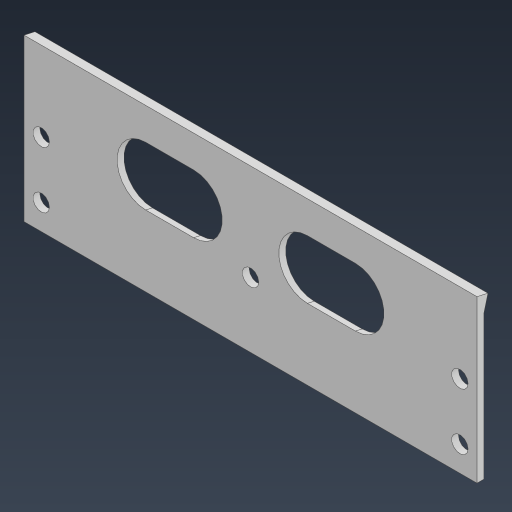
# Autodesk Inventor part: plastic_front
Saved by Autodesk Inventor 2023 (Build 270158000, 158)
## iProperties
Created: 2026-01-11
Part Number: plastic_front
Material: Generic
Document SubType Name: Modeling
Designer: szymo
Density: 14.3899 g/cm^3
Appearance: Default
Mass: 65 g
Surface Area: 65.7357 cm^2
Volume: 4.51705 cm^3
Author: szymo
Autodesk Inventor part; units mm, degrees
ref_plane "YZ Plane" through (0, 0, 0) normal (1, 0, 0) x (0, 1, 0)
ref_plane "XZ Plane" through (0, 0, 0) normal (0, 1, 0) x (-1, 0, 0)
ref_plane "XY Plane" through (0, 0, 0) normal (0, 0, 1) x (1, 0, 0)
ref_plane "Work Plane1" through (0, -9.9648, -37.8181) normal (-1, 0, 0) x (0, 0.2547957, 0.9669949)
sketch "Sketch1" plane through (0, -9.9648, -37.8181) normal (-1, 0, 0) x (0, 0.2547957, 0.9669949)
  line L0 (39.1088, 0) -> (31.1137, -30.3429) projected
  line L1 (0, 0) -> (39.1088, 0) projected
  line L2 (0, 0) -> (0, -30.3429) projected
  line L3 (31.1137, -30.3429) -> (0, -30.3429) projected
  line L4 (39.1088, 0) -> (40.5593, -0.3822)
  line L5 (40.5593, -0.3822) -> (32.5642, -30.7251)
  line L6 (32.5642, -30.7251) -> (31.1137, -30.3429)
  line L7 (41.4807, -0.7885) -> (33.5258, -30.9785) construction
  line L8 (33.5258, -30.9785) -> (32.5642, -30.7251) construction
  circle A0 centre (45.1128, -1.7455) radius 3.7561 construction
  line L9 (45.1128, 2.0106) -> (43.6538, 2.0106) construction
  line L10 (45.1128, 2.0106) -> (45.1128, -1.7455) construction
  circle A1 centre (-26.5758, -13.5) radius 17.5
  circle A2 centre (-26.5758, -13.5) radius 20
  line L11 (-26.5758, -13.5) -> (-26.5758, 6.5)
  line L12 (-26.5758, 6.5) -> (39.1088, 4)
  line L13 (40.5593, -0.3822) -> (41.6881, 3.9018)
  line L14 (39.1088, 4) -> (41.6881, 3.9018)
  line L15 (39.1088, 0) -> (39.1088, 4)
  line L16 (41.5576, 3.4064) -> (39.1088, 3.4996)
  dimension "d14" = 40
  dimension "d17" = 7.5122
  dimension "d0" = 1.5
  dimension "d16" = 180
  dimension "d18" = 0.5
  constraints: 26 end point, 4 vertical, 3 horizontal, 3 parallel, 2 perpendicular, 2 point on line, 1 centre point, 1 coincident, 1 collinear, 1 vertical alignment, 10 other
  measures "d0" distance between parallel lines of L0 L5
  measures "d16" angle of L14 L12
  measures "d18" distance between parallel lines of L14 L16
ref_plane "Work Plane2" through (99, -39.3062, -37.8181) normal (1, 0, 0) x (0, 0.9669949, -0.2547957)
extrude "Extrusion1" add sketch "Sketch1" against normal up to surface (99 mm away) contours L4 L5 L6 L0 | L15 L16 L13 L4
sketch "Sketch2" plane through (0, -31.3786, 1.5) normal (0, 0, 1) x (1, 0, 0)
  circle A0 centre (3.75, 17.8786) radius 2.75 projected
  circle A1 centre (3.75, 5.5) radius 2.75 projected
  line L0 (13.475, 24.7459) -> (13.475, 17.9349) projected
  line L1 (18.3, 24.7459) -> (13.475, 24.7459) projected
  line L2 (18.3, 24.7459) -> (18.3, 30.603) projected
  line L3 (3.625, 30.603) -> (18.3, 30.603) projected
  line L4 (3.625, 31.3786) -> (3.625, 30.603) projected
  line L5 (0, 31.3786) -> (3.625, 31.3786) projected
  line L6 (0, 31.3786) -> (0, 0) projected
  line L7 (0, 0) -> (7.5, 0) projected
  line L8 (7.5, 0) -> (7.5, 17.9349) projected
  line L9 (7.5, 17.9349) -> (13.475, 17.9349) projected
  circle A2 centre (95.25, 17.8786) radius 2.75 projected
  circle A3 centre (95.25, 5.5) radius 2.75 projected
  line L10 (85.525, 24.7459) -> (85.525, 17.9349) projected
  line L11 (91.5, 17.9349) -> (85.525, 17.9349) projected
  line L12 (91.5, 0) -> (91.5, 17.9349) projected
  line L13 (99, 0) -> (91.5, 0) projected
  line L14 (99, 31.3786) -> (99, 0) projected
  line L15 (99, 31.3786) -> (95.375, 31.3786) projected
  line L16 (95.375, 31.3786) -> (95.375, 30.603) projected
  line L17 (95.375, 30.603) -> (80.7, 30.603) projected
  line L18 (80.7, 24.7459) -> (80.7, 30.603) projected
  line L19 (80.7, 24.7459) -> (85.525, 24.7459) projected
  circle A4 centre (49.5, 14.1959) radius 2.25 projected
  constraints: 5 coincident
hole "Hole1" at (95.25, -25.8786, 1.5) at (95.25, -13.5, 1.5) at (3.75, -13.5, 1.5) at (3.75, -25.8786, 1.5) at (49.5, -17.1826, 1.5) direction (0, 0, -1) diameter 3.6 end through all clearance for "Countersunk Flat Head Screw ISO 2009/7046" size "M3" standard "ISO"
ref_plane "Work Plane3" through (67.175, -2.8957, 32.2865) normal (0, 0.224296, 0.9745211) x (-1, 0, 0)
sketch "Sketch3" plane through (67.175, -2.8957, 32.2865) normal (0, 0.224296, 0.9745211) x (-1, 0, 0)
  line L0 (-12.325, 5.5) -> (-12.325, -4.5) projected
  arc A0 (-12.325, -4.5) -> (-8.325, -8.5) centre (-8.325, -4.5) ccw projected
  line L1 (-8.325, -8.5) -> (8.325, -8.5) projected
  arc A1 (8.325, -8.5) -> (12.325, -4.5) centre (8.325, -4.5) ccw projected
  line L2 (12.325, -4.5) -> (12.325, 5.5) projected
  arc A2 (12.325, 5.5) -> (9.325, 8.5) centre (9.325, 5.5) ccw projected
  line L3 (9.325, 8.5) -> (-9.325, 8.5) projected
  arc A3 (-9.325, 8.5) -> (-12.325, 5.5) centre (-9.325, 5.5) ccw projected
  arc A4 (0, -0.2709) -> (0, -0.7291) centre (-5.245, -0.5) ccw projected
  arc A5 (0, -0.7291) -> (0, -0.2709) centre (5.245, -0.5) ccw projected
  line L4 (23.025, 5.5) -> (23.025, -4.5) projected
  arc A6 (23.025, -4.5) -> (27.025, -8.5) centre (27.025, -4.5) ccw projected
  line L5 (27.025, -8.5) -> (43.675, -8.5) projected
  arc A7 (43.675, -8.5) -> (47.675, -4.5) centre (43.675, -4.5) ccw projected
  line L6 (47.675, -4.5) -> (47.675, 5.5) projected
  arc A8 (47.675, 5.5) -> (44.675, 8.5) centre (44.675, 5.5) ccw projected
  line L7 (44.675, 8.5) -> (26.025, 8.5) projected
  arc A9 (26.025, 8.5) -> (23.025, 5.5) centre (26.025, 5.5) ccw projected
  arc A10 (35.35, -0.2709) -> (35.35, -0.7291) centre (30.105, -0.5) ccw projected
  arc A11 (35.35, -0.7291) -> (35.35, -0.2709) centre (40.595, -0.5) ccw projected
  line L8 (-5.245, -0.5) -> (5.245, -0.5) construction
  line L9 (-5.245, -5.75) -> (5.245, -5.75)
  line L10 (5.245, 4.75) -> (-5.245, 4.75)
  arc A12 (-5.245, 4.75) -> (-5.245, -5.75) centre (-5.245, -0.5) ccw
  arc A13 (5.245, -5.75) -> (5.245, 4.75) centre (5.245, -0.5) ccw
  line L11 (30.105, -0.5) -> (40.595, -0.5) construction
  line L12 (30.105, -5.75) -> (40.595, -5.75)
  line L13 (40.595, 4.75) -> (30.105, 4.75)
  arc A14 (30.105, 4.75) -> (30.105, -5.75) centre (30.105, -0.5) ccw
  arc A15 (40.595, -5.75) -> (40.595, 4.75) centre (40.595, -0.5) ccw
  line L14 (-5.245, 5.75) -> (5.245, 5.75)
  arc A16 (5.245, -6.75) -> (5.245, 5.75) centre (5.245, -0.5) ccw
  line L15 (5.245, -6.75) -> (-5.245, -6.75)
  arc A17 (-5.245, 5.75) -> (-5.245, -6.75) centre (-5.245, -0.5) ccw
  line L16 (30.105, 5.75) -> (40.595, 5.75)
  arc A18 (40.595, -6.75) -> (40.595, 5.75) centre (40.595, -0.5) ccw
  line L17 (40.595, -6.75) -> (30.105, -6.75)
  arc A19 (30.105, 5.75) -> (30.105, -6.75) centre (30.105, -0.5) ccw
  point P0 (67.175, -10.0637)
  point P1 (0, -0.5)
  point P2 (35.35, -0.5)
  dimension "d10" = 1
  dimension "d11" = 1
  constraints: 24 end point, 16 point on circle, 9 tangent, 8 centre point, 5 parallel, 2 midpoint, 1 concentric, 1 horizontal, 6 other
  measures "d10" distance between parallel lines of L10 L14
  measures "d11" distance between parallel lines of L13 L16
extrude "Extrusion2" cut sketch "Sketch3" against normal up to next contours A5 A4 | A4 L10 A5 | A4 A5 L9 | A11 A10 | A10 L13 A11 | A10 A11 L12 | L14 A16 L15 A17 | L16 A18 L17 A19
body "Solid1"
